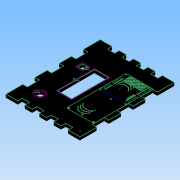
# Autodesk Inventor part: LCDWall
Saved by Autodesk Inventor 2015 (Build 190159000, 159)
## iProperties
Created: 2014-11-11
Part Number: LCDWall
Material: Generic
Document SubType Name: Modeling
Designer: 0
Density: 1 g/cm^3
Appearance: Plywood - Weathered
Mass: 139.736 g
Surface Area: 525.879 cm^2
Volume: 139.736 cm^3
Author: 0
Autodesk Inventor part; units mm, degrees
(part 1 of 2)
ref_plane "YZ Plane" through (0, 0, 0) normal (1, 0, 0) x (0, 1, 0)
ref_plane "XZ Plane" through (0, 0, 0) normal (0, 1, 0) x (-1, 0, 0)
ref_plane "XY Plane" through (0, 0, 0) normal (0, 0, 1) x (1, 0, 0)
sketch "Sketch1" plane through (0, 0, 0) normal (0, 1, 0) x (-1, 0, 0)
  line L0 (0, 0) -> (127, 0)
  line L1 (127, 0) -> (127, -166.624)
  line L2 (127, -166.624) -> (0, -166.624)
  line L3 (0, -166.624) -> (0, 0)
  dimension "BoxHeight" = 127
  dimension "d1" = 166.624
  constraints: 8 end point, 2 parallel, 1 coincident, 1 horizontal, 1 perpendicular
  measures "BoxHeight" distance of L1.end L2.end
  measures "d1" distance of L0.end L1.end
sketch "Sketch2" plane through (0, 0, 0) normal (0, 1, 0) x (-1, 0, 0)
  line L0 (0, 0) -> (-8.89, 0)
  line L1 (-8.89, 0) -> (-8.89, -23.8034)
  line L2 (-8.89, -23.8034) -> (0, -23.8034)
  line L3 (0, -23.8034) -> (0, 0)
  line L4 (0, -166.624) -> (0, 0) projected
  line L5 (0, 0) -> (127, 0) projected
  line L6 (0, -47.6069) -> (-8.89, -47.6069)
  line L7 (-8.89, -47.6069) -> (-8.89, -71.4103)
  line L8 (-8.89, -71.4103) -> (0, -71.4103)
  line L9 (0, -71.4103) -> (0, -47.6069)
  line L10 (0, -95.2137) -> (-8.89, -95.2137)
  line L11 (-8.89, -95.2137) -> (-8.89, -119.0171)
  line L12 (-8.89, -119.0171) -> (0, -119.0171)
  line L13 (0, -119.0171) -> (0, -95.2137)
  line L14 (63.5, 0) -> (63.5, -115.824) construction
  line L15 (127, -23.8034) -> (127, 0)
  line L16 (127, -166.624) -> (127, 0)
  line L17 (127, -71.4103) -> (127, -47.6069)
  line L18 (127, -119.0171) -> (127, -95.2137)
  line L19 (28.2222, -166.624) -> (14.1111, -166.624)
  line L20 (14.1111, -166.624) -> (14.1111, -175.514)
  line L21 (14.1111, -175.514) -> (28.2222, -175.514)
  line L22 (28.2222, -175.514) -> (28.2222, -166.624)
  line L23 (127, -166.624) -> (0, -166.624) projected
  line L24 (56.4444, -166.624) -> (42.3333, -166.624)
  line L25 (42.3333, -166.624) -> (42.3333, -175.514)
  line L26 (42.3333, -175.514) -> (56.4444, -175.514)
  line L27 (56.4444, -175.514) -> (56.4444, -166.624)
  line L28 (84.6667, -166.624) -> (70.5556, -166.624)
  line L29 (70.5556, -166.624) -> (70.5556, -175.514)
  line L30 (70.5556, -175.514) -> (84.6667, -175.514)
  line L31 (84.6667, -175.514) -> (84.6667, -166.624)
  line L32 (112.8889, -166.624) -> (98.7778, -166.624)
  line L33 (98.7778, -166.624) -> (98.7778, -175.514)
  line L34 (98.7778, -175.514) -> (112.8889, -175.514)
  line L35 (112.8889, -175.514) -> (112.8889, -166.624)
  line L36 (127, -83.312) -> (0, -83.312) construction
  line L37 (63.5, -166.624) -> (63.5, -50.8) construction
  line L38 (28.2222, 0) -> (14.1111, 0)
  line L39 (14.1111, 0) -> (14.1111, 8.89)
  line L40 (14.1111, 8.89) -> (28.2222, 8.89)
  line L41 (28.2222, 8.89) -> (28.2222, 0)
  line L42 (127, 0) -> (0, 0)
  line L43 (56.4444, 0) -> (42.3333, 0)
  line L44 (42.3333, 0) -> (42.3333, 8.89)
  line L45 (42.3333, 8.89) -> (56.4444, 8.89)
  line L46 (56.4444, 8.89) -> (56.4444, 0)
  line L47 (84.6667, 0) -> (70.5556, 0)
  line L48 (70.5556, 0) -> (70.5556, 8.89)
  line L49 (84.6667, 8.89) -> (84.6667, 0)
  line L50 (70.5556, 8.89) -> (84.6667, 8.89)
  line L51 (112.8889, 0) -> (98.7778, 0)
  line L52 (98.7778, 0) -> (98.7778, 8.89)
  line L53 (112.8889, 8.89) -> (112.8889, 0)
  line L54 (98.7778, 8.89) -> (112.8889, 8.89)
  line L55 (0, -142.8206) -> (-8.89, -142.8206)
  line L56 (-8.89, -142.8206) -> (-8.89, -159.3669)
  line L57 (-8.89, -159.3669) -> (0, -159.3669)
  line L58 (0, -159.3669) -> (0, -142.8206)
  line L59 (127, -166.624) -> (127, 0)
  line L60 (127, 0) -> (135.89, 0)
  line L61 (135.89, 0) -> (135.89, -23.8034)
  line L62 (135.89, -23.8034) -> (127, -23.8034)
  line L63 (127, -23.8034) -> (127, 0)
  line L64 (127, -166.624) -> (127, 0)
  line L65 (127, -47.6069) -> (135.89, -47.6069)
  line L66 (135.89, -47.6069) -> (135.89, -71.4103)
  line L67 (135.89, -71.4103) -> (127, -71.4103)
  line L68 (127, -71.4103) -> (127, -47.6069)
  line L69 (127, -95.2137) -> (135.89, -95.2137)
  line L70 (135.89, -95.2137) -> (135.89, -119.0171)
  line L71 (135.89, -119.0171) -> (127, -119.0171)
  line L72 (127, -119.0171) -> (127, -95.2137)
  line L73 (135.89, -142.8206) -> (135.89, -159.3669)
  line L74 (127, -142.8206) -> (135.89, -142.8206)
  line L75 (127, -159.3669) -> (127, -142.8206)
  line L76 (135.89, -159.3669) -> (127, -159.3669)
  line L77 (14.1111, -175.514) -> (0, -175.514)
  line L78 (0, -175.514) -> (0, -159.3669)
  line L79 (0, -159.3669) -> (14.1111, -159.3669)
  line L80 (14.1111, -159.3669) -> (14.1111, -175.514)
  line L81 (28.2222, -175.514) -> (42.3333, -175.514)
  line L82 (42.3333, -175.514) -> (42.3333, -166.624)
  line L83 (42.3333, -166.624) -> (28.2222, -166.624)
  line L84 (28.2222, -166.624) -> (28.2222, -175.514)
  line L85 (56.4444, -175.514) -> (70.5556, -175.514)
  line L86 (70.5556, -175.514) -> (70.5556, -166.624)
  line L87 (70.5556, -166.624) -> (56.4444, -166.624)
  line L88 (56.4444, -166.624) -> (56.4444, -175.514)
  line L89 (84.6667, -175.514) -> (98.7778, -175.514)
  line L90 (98.7778, -175.514) -> (98.7778, -166.624)
  line L91 (98.7778, -166.624) -> (84.6667, -166.624)
  line L92 (84.6667, -166.624) -> (84.6667, -175.514)
  line L93 (112.8889, -175.514) -> (127, -175.514)
  line L94 (127, -175.514) -> (127, -159.3669)
  line L95 (127, -159.3669) -> (112.8889, -159.3669)
  line L96 (112.8889, -159.3669) -> (112.8889, -175.514)
  line L97 (112.8889, 0) -> (127, 0)
  line L98 (127, 0) -> (127, 8.89)
  line L99 (127, 8.89) -> (112.8889, 8.89)
  line L100 (112.8889, 8.89) -> (112.8889, 0)
  line L101 (98.7778, 8.89) -> (84.6667, 8.89)
  line L102 (84.6667, 8.89) -> (84.6667, 0)
  line L103 (84.6667, 0) -> (98.7778, 0)
  line L104 (98.7778, 0) -> (98.7778, 8.89)
  line L105 (70.5556, 8.89) -> (56.4444, 8.89)
  line L106 (56.4444, 8.89) -> (56.4444, 0)
  line L107 (56.4444, 0) -> (70.5556, 0)
  line L108 (70.5556, 0) -> (70.5556, 8.89)
  line L109 (42.3333, 8.89) -> (28.2222, 8.89)
  line L110 (28.2222, 8.89) -> (28.2222, 0)
  line L111 (28.2222, 0) -> (42.3333, 0)
  line L112 (42.3333, 0) -> (42.3333, 8.89)
  line L113 (14.1111, 8.89) -> (0, 8.89)
  line L114 (0, 8.89) -> (0, 0)
  line L115 (0, 0) -> (14.1111, 0)
  line L116 (14.1111, 0) -> (14.1111, 8.89)
  line L117 (0, 0) -> (-8.89, 0)
  line L118 (-8.89, 0) -> (-8.89, 8.89)
  line L119 (-8.89, 8.89) -> (0, 8.89)
  line L120 (0, 8.89) -> (0, 0)
  line L121 (0, -159.3669) -> (-8.89, -159.3669)
  line L122 (-8.89, -159.3669) -> (-8.89, -168.2569)
  line L123 (-8.89, -168.2569) -> (0, -168.2569)
  line L124 (0, -168.2569) -> (0, -159.3669)
  line L125 (127, -159.3669) -> (135.89, -159.3669)
  line L126 (135.89, -159.3669) -> (135.89, -168.2569)
  line L127 (135.89, -168.2569) -> (127, -168.2569)
  line L128 (127, -168.2569) -> (127, -159.3669)
  line L129 (127, 0) -> (135.89, 0)
  line L130 (135.89, 0) -> (135.89, 8.89)
  line L131 (135.89, 8.89) -> (127, 8.89)
  line L132 (127, 8.89) -> (127, 0)
  line L133 (135.89, -168.2569) -> (127, -168.2569)
  line L134 (127, -168.2569) -> (127, -175.514)
  line L135 (127, -175.514) -> (135.89, -175.514)
  line L136 (135.89, -175.514) -> (135.89, -168.2569)
  line L137 (0, -175.514) -> (-8.89, -175.514)
  line L138 (-8.89, -175.514) -> (-8.89, -168.2569)
  line L139 (-8.89, -168.2569) -> (0, -168.2569)
  line L140 (0, -168.2569) -> (0, -175.514)
  dimension "d2" = 8.89
  dimension "d3" = 23.8034
  dimension "d5" = 8.89
  dimension "d6" = 23.8034
  dimension "d7" = 23.8034
  dimension "d8" = 8.89
  dimension "d9" = 23.8034
  dimension "d10" = 23.8034
  dimension "d11" = 14.1111
  dimension "d12" = 127
  dimension "d13" = 14.1111
  dimension "d14" = 8.89
  dimension "d15" = 8.89
  dimension "d16" = 14.1111
  dimension "d17" = 8.89
  dimension "d18" = 14.1111
  dimension "d22" = 8.89
  dimension "d23" = 14.1111
  dimension "d27" = 14.1111
  dimension "d28" = 14.1111
  dimension "d29" = 14.1111
  dimension "d34" = 8.89
  dimension "d35" = 16.5463
  dimension "d40" = 23.8034
  dimension "d41" = 8.89
  dimension "d42" = 8.89
  dimension "d43" = 8.89
  dimension "d44" = 8.89
  dimension "d45" = 8.89
  dimension "d46" = 8.89
  dimension "d47" = 8.89
  dimension "d48" = 8.89
  constraints: 276 end point, 48 parallel, 43 symmetric about line, 24 horizontal, 24 perpendicular, 9 collinear, 2 midpoint, 1 point on line, 1 vertical
  measures "d2" distance of L1.end L2.end
  measures "d3" distance of L0.end L1.end
  measures "d5" distance of L7.end L8.end
  measures "d6" distance of L6.end L7.end
  measures "d7" distance between parallel lines of L2 L6
  measures "d8" distance of L10.start L10.end
  measures "d9" distance of L10.end L11.end
  measures "d10" distance between parallel lines of L8 L10
  measures "d11" distance between parallel lines of L4 L20
  measures "d12" distance of L23.start L4.start
  measures "d13" distance of L20.end L21.end
  measures "d14" distance of L19.end L20.end
  measures "d15" distance of L24.end L25.end
  measures "d16" distance of L25.end L26.end
  measures "d17" distance of L28.end L29.end
  measures "d18" distance of L29.end L31.start
  measures "d22" distance of L32.end L33.end
  measures "d23" distance of L33.end L35.start
  measures "d27" distance between parallel lines of L25 L22
  measures "d28" distance between parallel lines of L27 L29
  measures "d29" distance between parallel lines of L31 L33
  measures "d34" distance of L55.start L56.start
  measures "d35" distance of L56.start L56.end
  measures "d40" distance between parallel lines of L12 L55
  measures "d41" distance of L118.end L119.end
  measures "d42" distance of L117.end L118.end
  measures "d43" distance of L123.end L122.end
  measures "d44" distance of L122.end L121.end
  measures "d45" distance of L126.end L127.end
  measures "d46" distance of L125.end L126.end
  measures "d47" distance of L131.end L130.end
  measures "d48" distance of L130.end L129.end
extrude "Connections" add sketch "Sketch2" along normal blind 6.35 contours L3 L2 L1 L0 | L114 L113 L39 L5 | L0 L118 L119 L114 | L4 L8 L7 L6 | L41 L109 L44 L5 | L4 L12 L11 L10 | L46 L105 L48 L5 | L4 L57 L56 L55 | L49 L101 L52 L5 | L79 L80 L23 L4 | L4 L78 L123 L122 L57 | L23 L20 L77 L78 | L53 L99 L98 L5 | L78 L137 L138 L123 | L60 L61 L62 L15 | L98 L131 L130 L60 | L23 L25 L81 L22 | L65 L66 L67 L16 | L23 L29 L85 L27 | L69 L70 L71 L16 | L23 L33 L89 L31 | L74 L73 L76 L16 | L96 L95 L16 L23 | L23 L94 L93 L35 | L76 L126 L127 L94 L16 | L94 L127 L136 L135
extrude "Base Extrusion" add sketch "Sketch1" along normal blind 6.35
sketch "Sketch3" plane through (0, 0, 0) normal (0, -1, 0) x (1, 0, 0)
  line L0 (-70.5556, 8.89) -> (-56.4444, 8.89) projected
  line L1 (-63.5, 8.89) -> (-63.5, -175.514) construction
  line L2 (-56.4444, -175.514) -> (-70.5556, -175.514) projected
  line L3 (8.89, -83.312) -> (-135.89, -83.312) construction
  line L4 (-28.2222, -175.514) -> (-42.3333, -175.514) projected
  line L5 (-42.3333, 8.89) -> (-28.2222, 8.89) projected
  line L6 (8.89, -175.514) -> (8.89, -142.8206) projected
  line L7 (-135.89, -175.514) -> (-135.89, -142.8206) projected
  line L8 (-135.89, -119.0171) -> (-135.89, -95.2137) projected
  line L9 (-91.186, -47.117) -> (-63.5, -47.117)
  line L10 (-63.5, -47.117) -> (-63.5, -119.507)
  line L11 (-63.5, -119.507) -> (-91.186, -119.507)
  line L12 (-91.186, -119.507) -> (-91.186, -47.117)
  point P0 (0, 0)
  point P1 (8.89, -168.2569)
  point P2 (-135.89, -168.2569)
  dimension "d49" = 184.404
  dimension "d50" = 92.202
  dimension "d51" = 144.78
  dimension "d52" = 144.78
  dimension "d53" = 0
  dimension "d54" = 27.686
  dimension "d55" = 72.39
  dimension "d56" = 27.686
  dimension "d57" = 36.195
  constraints: 12 end point, 2 horizontal, 2 midpoint, 2 parallel, 1 perpendicular
  measures "d49" distance between parallel lines of L4 L5
  measures "d50" distance between parallel lines of L4 L3
  measures "d51" distance between parallel lines of L6 L7
  measures "d52" distance of L3.start L3.end
  measures "d53" distance from line of L8 L3.end
  measures "d54" distance of L10.end L11.end
  measures "d55" distance of L11.end L9.start
  measures "d56" distance between parallel lines of L1 L12
  measures "d57" distance between parallel lines of L3 L9
extrude "LCD Hole" cut sketch "Sketch3" against normal blind 25.4
sketch "Sketch5" plane through (0, 0, 0) normal (0, -1, 0) x (1, 0, 0)
  line L0 (-3.8506, -48.6761) -> (-3.8506, -68.028) construction
  line L1 (-3.8506, -68.028) -> (-44.1343, -68.028) construction
  line L2 (-44.1343, -68.028) -> (-44.1343, -48.6761) construction
  line L3 (-44.1343, -48.6761) -> (-3.8506, -48.6761) construction
  point P0 (0, 0)
  constraints: 2 other
sketch "Sketch7" plane through (0, 6.35, 0) normal (0, 1, 0) x (1, 0, 0)
  circle A0 centre (-102.8514, 25.0329) radius 6.985 projected
  point P0 (0, 0)
extrude "Extrusion4" cut sketch "Sketch7" against normal blind 25.4
sketch "Sketch6" plane through (0, 6.35, 0) normal (0, 1, 0) x (1, 0, 0)
  arc A0 (-44.8569, 41.3319) -> (-21.0385, 41.4572) centre (-32.9709, 45.8056) ccw
  arc A1 (-44.9033, 46.638) -> (-21.0849, 46.5126) centre (-32.9709, 50.9863) ccw
  arc A2 (-44.8569, 51.4366) -> (-21.0849, 51.4366) centre (-32.9709, 55.9103) ccw
  line L0 (-21.0385, 41.4572) -> (-44.9033, 41.4572) construction
  line L1 (-44.9033, 41.4572) -> (-44.9033, 76.962) construction
  line L2 (-44.9033, 76.962) -> (-21.0385, 76.962) construction
  line L3 (-21.0385, 76.962) -> (-21.0385, 41.4572) construction
  line L4 (-63.5, 47.117) -> (-2.4418, 47.117) construction
  line L5 (-2.4418, 47.117) -> (-2.4418, 119.507) construction
  line L6 (-2.4418, 119.507) -> (-63.5, 119.507) construction
  line L7 (-63.5, 119.507) -> (-63.5, 47.117) construction
  line L8 (-2.4418, 83.312) -> (-63.5, 83.312) construction
  line L9 (-63.5, 47.117) -> (-63.5, 119.507) projected
  line L10 (-32.9709, 47.117) -> (-32.9709, 119.507) construction
  line L11 (-46.2663, 76.962) -> (-23.7437, 76.962) construction
  line L12 (-21.5465, 41.5479) -> (-21.5465, 51.054) construction
  arc A3 (-44.3611, 46.638) -> (-21.6293, 46.5126) centre (-32.9709, 50.9863) ccw
  arc A4 (-44.3125, 51.4366) -> (-21.6293, 51.4366) centre (-32.9709, 55.9103) ccw
  line L13 (-21.5465, 51.054) -> (-21.5465, 41.5479) construction
  line L14 (-44.8569, 41.3319) -> (-44.3125, 41.3319)
  arc A5 (-44.3125, 41.3319) -> (-21.5807, 41.4572) centre (-32.9709, 45.8056) ccw
  line L15 (-21.0385, 41.4572) -> (-21.5807, 41.4572)
  line L16 (-21.0849, 46.5126) -> (-21.6293, 46.5126)
  line L17 (-21.0849, 51.4366) -> (-21.6293, 51.4366)
  line L18 (-44.9033, 46.638) -> (-44.3611, 46.638)
  line L19 (-44.3611, 76.962) -> (-44.9033, 76.962)
  line L20 (-21.6293, 51.4366) -> (4.4309, 51.4366) construction
  line L21 (-44.3125, 51.4366) -> (-44.8569, 51.4366)
  arc A6 (-21.0385, 125.1668) -> (-44.8569, 125.2921) centre (-32.9709, 120.8184) ccw
  arc A7 (-21.0849, 120.1114) -> (-44.9033, 119.986) centre (-32.9709, 115.6377) ccw
  arc A8 (-21.0849, 115.1874) -> (-44.8569, 115.1874) centre (-32.9709, 110.7137) ccw
  line L22 (-21.0385, 125.1668) -> (-44.9033, 125.1668) construction
  line L23 (-44.9033, 125.1668) -> (-44.9033, 89.662) construction
  line L24 (-44.9033, 89.662) -> (-21.0385, 89.662) construction
  line L25 (-21.0385, 89.662) -> (-21.0385, 125.1668) construction
  line L26 (-32.9709, 119.507) -> (-32.9709, 47.117) construction
  line L27 (-46.2663, 89.662) -> (-23.7437, 89.662) construction
  line L28 (-21.5465, 125.0761) -> (-21.5465, 115.57) construction
  arc A9 (-21.6293, 120.1114) -> (-44.3611, 119.986) centre (-32.9709, 115.6377) ccw
  arc A10 (-21.6293, 115.1874) -> (-44.3125, 115.1874) centre (-32.9709, 110.7137) ccw
  line L29 (-21.5465, 115.57) -> (-21.5465, 125.0761) construction
  line L30 (-44.8569, 125.2921) -> (-44.3125, 125.2921)
  arc A11 (-21.5807, 125.1668) -> (-44.3125, 125.2921) centre (-32.9709, 120.8184) ccw
  line L31 (-21.0385, 125.1668) -> (-21.5807, 125.1668)
  line L32 (-21.0849, 120.1114) -> (-21.6293, 120.1114)
  line L33 (-21.0849, 115.1874) -> (-21.6293, 115.1874)
  line L34 (-44.9033, 119.986) -> (-44.3611, 119.986)
  line L35 (-44.3611, 89.662) -> (-44.9033, 89.662)
  line L36 (-21.6293, 115.1874) -> (4.4309, 115.1874) construction
  line L37 (-44.3125, 115.1874) -> (-44.8569, 115.1874)
  line L38 (-0.1825, 29.2815) -> (-0.1825, 141.0415) projected
  arc A12 (-2.7225, 26.7415) -> (-0.1825, 29.2815) centre (-2.7225, 29.2815) ccw projected
  line L39 (-50.9825, 26.7415) -> (-2.7225, 26.7415) projected
  arc A13 (-53.5225, 29.2815) -> (-50.9825, 26.7415) centre (-50.9825, 29.2815) ccw projected
  line L40 (-53.5225, 141.0415) -> (-53.5225, 29.2815) projected
  arc A14 (-50.9825, 143.5815) -> (-53.5225, 141.0415) centre (-50.9825, 141.0415) ccw projected
  line L41 (-2.7225, 143.5815) -> (-50.9825, 143.5815) projected
  arc A15 (-0.1825, 141.0415) -> (-2.7225, 143.5815) centre (-2.7225, 141.0415) ccw projected
  line L42 (-2.405, 141.994) -> (-2.405, 141.359) projected
  line L43 (-3.04, 141.994) -> (-2.405, 141.994) projected
  line L44 (-3.04, 141.359) -> (-3.04, 141.994) projected
  line L45 (-2.405, 141.359) -> (-3.04, 141.359) projected
  line L46 (-50.665, 127.389) -> (-50.665, 126.754) projected
  line L47 (-51.3, 127.389) -> (-50.665, 127.389) projected
  line L48 (-51.3, 126.754) -> (-51.3, 127.389) projected
  line L49 (-50.665, 126.754) -> (-51.3, 126.754) projected
  line L50 (-50.665, 122.309) -> (-50.665, 121.674) projected
  line L51 (-51.3, 122.309) -> (-50.665, 122.309) projected
  line L52 (-51.3, 121.674) -> (-51.3, 122.309) projected
  line L53 (-50.665, 121.674) -> (-51.3, 121.674) projected
  line L54 (-50.665, 117.229) -> (-50.665, 116.594) projected
  line L55 (-51.3, 117.229) -> (-50.665, 117.229) projected
  line L56 (-51.3, 116.594) -> (-51.3, 117.229) projected
  line L57 (-50.665, 116.594) -> (-51.3, 116.594) projected
  line L58 (-50.665, 109.609) -> (-50.665, 108.974) projected
  line L59 (-51.3, 109.609) -> (-50.665, 109.609) projected
  line L60 (-51.3, 108.974) -> (-51.3, 109.609) projected
  line L61 (-50.665, 108.974) -> (-51.3, 108.974) projected
  line L62 (-50.665, 104.529) -> (-50.665, 103.894) projected
  line L63 (-51.3, 104.529) -> (-50.665, 104.529) projected
  line L64 (-51.3, 103.894) -> (-51.3, 104.529) projected
  line L65 (-50.665, 103.894) -> (-51.3, 103.894) projected
  line L66 (-50.665, 99.449) -> (-50.665, 98.814) projected
  line L67 (-51.3, 99.449) -> (-50.665, 99.449) projected
  line L68 (-51.3, 98.814) -> (-51.3, 99.449) projected
  line L69 (-50.665, 98.814) -> (-51.3, 98.814) projected
  line L70 (-2.405, 115.324) -> (-2.405, 114.689) projected
  line L71 (-3.04, 115.324) -> (-2.405, 115.324) projected
  line L72 (-3.04, 114.689) -> (-3.04, 115.324) projected
  line L73 (-2.405, 114.689) -> (-3.04, 114.689) projected
  line L74 (-3.04, 136.914) -> (-2.405, 136.914) projected
  line L75 (-3.04, 136.279) -> (-3.04, 136.914) projected
  line L76 (-2.405, 136.279) -> (-3.04, 136.279) projected
  line L77 (-2.405, 136.914) -> (-2.405, 136.279) projected
  line L78 (-3.04, 131.834) -> (-2.405, 131.834) projected
  line L79 (-3.04, 131.199) -> (-3.04, 131.834) projected
  line L80 (-2.405, 131.199) -> (-3.04, 131.199) projected
  line L81 (-2.405, 131.834) -> (-2.405, 131.199) projected
  line L82 (-3.04, 126.754) -> (-2.405, 126.754) projected
  line L83 (-3.04, 126.119) -> (-3.04, 126.754) projected
  line L84 (-2.405, 126.119) -> (-3.04, 126.119) projected
  line L85 (-2.405, 126.754) -> (-2.405, 126.119) projected
  line L86 (-3.04, 121.674) -> (-2.405, 121.674) projected
  line L87 (-3.04, 121.039) -> (-3.04, 121.674) projected
  line L88 (-2.405, 121.039) -> (-3.04, 121.039) projected
  line L89 (-2.405, 121.674) -> (-2.405, 121.039) projected
  line L90 (-2.405, 112.784) -> (-2.405, 112.149) projected
  line L91 (-3.04, 112.784) -> (-2.405, 112.784) projected
  line L92 (-3.04, 112.149) -> (-3.04, 112.784) projected
  line L93 (-2.405, 112.149) -> (-3.04, 112.149) projected
  line L94 (-2.405, 107.704) -> (-2.405, 107.069) projected
  line L95 (-3.04, 107.704) -> (-2.405, 107.704) projected
  line L96 (-3.04, 107.069) -> (-3.04, 107.704) projected
  line L97 (-2.405, 107.069) -> (-3.04, 107.069) projected
  line L98 (-2.405, 102.624) -> (-2.405, 101.989) projected
  line L99 (-3.04, 102.624) -> (-2.405, 102.624) projected
  line L100 (-3.04, 101.989) -> (-3.04, 102.624) projected
  line L101 (-2.405, 101.989) -> (-3.04, 101.989) projected
  line L102 (-2.405, 97.544) -> (-2.405, 96.909) projected
  line L103 (-3.04, 97.544) -> (-2.405, 97.544) projected
  line L104 (-3.04, 96.909) -> (-3.04, 97.544) projected
  line L105 (-2.405, 96.909) -> (-3.04, 96.909) projected
  circle A16 centre (-9.0725, 102.3065) radius 0.635 projected
  circle A17 centre (-9.0725, 104.8465) radius 0.635 projected
  circle A18 centre (-9.0725, 107.3865) radius 0.635 projected
  circle A19 centre (-9.0725, 109.9265) radius 0.635 projected
  circle A20 centre (-9.0725, 112.4665) radius 0.635 projected
  circle A21 centre (-9.0725, 115.0065) radius 0.635 projected
  circle A22 centre (-24.884, 29.9165) radius 0.3175 projected
  circle A23 centre (-26.535, 30.9325) radius 0.3175 projected
  circle A24 centre (-26.535, 32.9645) radius 0.3175 projected
  circle A25 centre (-23.36, 85.0345) radius 0.3175 projected
  circle A26 centre (-26.535, 86.0505) radius 0.3175 projected
  line L106 (-2.405, 100.084) -> (-2.405, 99.449) projected
  line L107 (-3.04, 100.084) -> (-2.405, 100.084) projected
  line L108 (-3.04, 99.449) -> (-3.04, 100.084) projected
  line L109 (-2.405, 99.449) -> (-3.04, 99.449) projected
  line L110 (-2.405, 105.164) -> (-2.405, 104.529) projected
  line L111 (-3.04, 105.164) -> (-2.405, 105.164) projected
  line L112 (-3.04, 104.529) -> (-3.04, 105.164) projected
  line L113 (-2.405, 104.529) -> (-3.04, 104.529) projected
  line L114 (-2.405, 110.244) -> (-2.405, 109.609) projected
  line L115 (-3.04, 110.244) -> (-2.405, 110.244) projected
  line L116 (-3.04, 109.609) -> (-3.04, 110.244) projected
  line L117 (-2.405, 109.609) -> (-3.04, 109.609) projected
  line L118 (-3.04, 119.134) -> (-2.405, 119.134) projected
  line L119 (-3.04, 118.499) -> (-3.04, 119.134) projected
  line L120 (-2.405, 118.499) -> (-3.04, 118.499) projected
  line L121 (-2.405, 119.134) -> (-2.405, 118.499) projected
  line L122 (-3.04, 124.214) -> (-2.405, 124.214) projected
  line L123 (-3.04, 123.579) -> (-3.04, 124.214) projected
  line L124 (-2.405, 123.579) -> (-3.04, 123.579) projected
  line L125 (-2.405, 124.214) -> (-2.405, 123.579) projected
  line L126 (-3.04, 129.294) -> (-2.405, 129.294) projected
  line L127 (-3.04, 128.659) -> (-3.04, 129.294) projected
  line L128 (-2.405, 128.659) -> (-3.04, 128.659) projected
  line L129 (-2.405, 129.294) -> (-2.405, 128.659) projected
  line L130 (-3.04, 134.374) -> (-2.405, 134.374) projected
  line L131 (-3.04, 133.739) -> (-3.04, 134.374) projected
  line L132 (-2.405, 133.739) -> (-3.04, 133.739) projected
  line L133 (-2.405, 134.374) -> (-2.405, 133.739) projected
  line L134 (-3.04, 139.454) -> (-2.405, 139.454) projected
  line L135 (-3.04, 138.819) -> (-3.04, 139.454) projected
  line L136 (-2.405, 138.819) -> (-3.04, 138.819) projected
  line L137 (-2.405, 139.454) -> (-2.405, 138.819) projected
  line L138 (-50.665, 96.909) -> (-50.665, 96.274) projected
  line L139 (-51.3, 96.909) -> (-50.665, 96.909) projected
  line L140 (-51.3, 96.274) -> (-51.3, 96.909) projected
  line L141 (-50.665, 96.274) -> (-51.3, 96.274) projected
  line L142 (-50.665, 101.989) -> (-50.665, 101.354) projected
  line L143 (-51.3, 101.989) -> (-50.665, 101.989) projected
  line L144 (-51.3, 101.354) -> (-51.3, 101.989) projected
  line L145 (-50.665, 101.354) -> (-51.3, 101.354) projected
  line L146 (-50.665, 107.069) -> (-50.665, 106.434) projected
  line L147 (-51.3, 107.069) -> (-50.665, 107.069) projected
  line L148 (-51.3, 106.434) -> (-51.3, 107.069) projected
  line L149 (-50.665, 106.434) -> (-51.3, 106.434) projected
  line L150 (-50.665, 114.689) -> (-50.665, 114.054) projected
  line L151 (-51.3, 114.689) -> (-50.665, 114.689) projected
  line L152 (-51.3, 114.054) -> (-51.3, 114.689) projected
  line L153 (-50.665, 114.054) -> (-51.3, 114.054) projected
  line L154 (-50.665, 119.769) -> (-50.665, 119.134) projected
  line L155 (-51.3, 119.769) -> (-50.665, 119.769) projected
  line L156 (-51.3, 119.134) -> (-51.3, 119.769) projected
  line L157 (-50.665, 119.134) -> (-51.3, 119.134) projected
  line L158 (-50.665, 124.849) -> (-50.665, 124.214) projected
  line L159 (-51.3, 124.849) -> (-50.665, 124.849) projected
  line L160 (-51.3, 124.214) -> (-51.3, 124.849) projected
  line L161 (-50.665, 124.214) -> (-51.3, 124.214) projected
  line L162 (-50.665, 129.929) -> (-50.665, 129.294) projected
  line L163 (-51.3, 129.929) -> (-50.665, 129.929) projected
  line L164 (-51.3, 129.294) -> (-51.3, 129.929) projected
  line L165 (-50.665, 129.294) -> (-51.3, 129.294) projected
  line L166 (-50.665, 132.469) -> (-50.665, 131.834) projected
  line L167 (-51.3, 132.469) -> (-50.665, 132.469) projected
  line L168 (-51.3, 131.834) -> (-51.3, 132.469) projected
  line L169 (-50.665, 131.834) -> (-51.3, 131.834) projected
  circle A27 centre (-47.1725, 96.5915) radius 0.635 projected
  circle A28 centre (-47.1725, 99.1315) radius 0.635 projected
  circle A29 centre (-47.1725, 101.6715) radius 0.635 projected
  circle A30 centre (-47.1725, 104.2115) radius 0.635 projected
  circle A31 centre (-47.1725, 106.7515) radius 0.635 projected
  circle A32 centre (-47.1725, 109.2915) radius 0.635 projected
  circle A33 centre (-47.1725, 114.3715) radius 0.635 projected
  circle A34 centre (-47.1725, 116.9115) radius 0.635 projected
  circle A35 centre (-47.1725, 119.4515) radius 0.635 projected
  circle A36 centre (-47.1725, 121.9915) radius 0.635 projected
  circle A37 centre (-47.1725, 124.5315) radius 0.635 projected
  circle A38 centre (-47.1725, 127.0715) radius 0.635 projected
  circle A39 centre (-47.1725, 129.6115) radius 0.635 projected
  circle A40 centre (-47.1725, 132.1515) radius 0.635 projected
  circle A41 centre (-6.5325, 97.2265) radius 0.635 projected
  circle A42 centre (-6.5325, 99.7665) radius 0.635 projected
  circle A43 centre (-6.5325, 102.3065) radius 0.635 projected
  circle A44 centre (-6.5325, 104.8465) radius 0.635 projected
  circle A45 centre (-6.5325, 107.3865) radius 0.635 projected
  circle A46 centre (-6.5325, 109.9265) radius 0.635 projected
  circle A47 centre (-6.5325, 112.4665) radius 0.635 projected
  circle A48 centre (-6.5325, 118.8165) radius 0.635 projected
  circle A49 centre (-6.5325, 121.3565) radius 0.635 projected
  circle A50 centre (-6.5325, 123.8965) radius 0.635 projected
  circle A51 centre (-6.5325, 126.4365) radius 0.635 projected
  circle A52 centre (-6.5325, 128.9765) radius 0.635 projected
  circle A53 centre (-6.5325, 131.5165) radius 0.635 projected
  circle A54 centre (-6.5325, 134.0565) radius 0.635 projected
  circle A55 centre (-6.5325, 136.5965) radius 0.635 projected
  circle A56 centre (-6.5325, 139.1365) radius 0.635 projected
  circle A57 centre (-6.5325, 115.0065) radius 0.635 projected
  circle A58 centre (-6.5325, 141.6765) radius 0.635 projected
  circle A59 centre (-10.3425, 141.6765) radius 0.635 projected
  circle A60 centre (-12.8825, 141.6765) radius 0.635 projected
  circle A61 centre (-15.4225, 141.6765) radius 0.635 projected
  circle A62 centre (-17.9625, 141.6765) radius 0.635 projected
  circle A63 centre (-20.5025, 141.6765) radius 0.635 projected
  circle A64 centre (-23.0425, 141.6765) radius 0.635 projected
  circle A65 centre (-25.5825, 141.6765) radius 0.635 projected
  circle A66 centre (-28.1225, 141.6765) radius 0.635 projected
  circle A67 centre (-30.6625, 141.6765) radius 0.635 projected
  circle A68 centre (-33.2025, 141.6765) radius 0.635 projected
  circle A69 centre (-35.7425, 141.6765) radius 0.635 projected
  circle A70 centre (-38.2825, 141.6765) radius 0.635 projected
  circle A71 centre (-40.8225, 141.6765) radius 0.635 projected
  circle A72 centre (-10.3425, 128.9765) radius 0.635 projected
  circle A73 centre (-10.3425, 131.5165) radius 0.635 projected
  circle A74 centre (-10.3425, 134.0565) radius 0.635 projected
  circle A75 centre (-10.3425, 136.5965) radius 0.635 projected
  circle A76 centre (-10.3425, 139.1365) radius 0.635 projected
  circle A77 centre (-12.8825, 128.9765) radius 0.635 projected
  circle A78 centre (-12.8825, 131.5165) radius 0.635 projected
  circle A79 centre (-12.8825, 134.0565) radius 0.635 projected
  circle A80 centre (-12.8825, 136.5965) radius 0.635 projected
  circle A81 centre (-12.8825, 139.1365) radius 0.635 projected
  circle A82 centre (-15.4225, 128.9765) radius 0.635 projected
  circle A83 centre (-15.4225, 131.5165) radius 0.635 projected
  circle A84 centre (-15.4225, 134.0565) radius 0.635 projected
  circle A85 centre (-15.4225, 136.5965) radius 0.635 projected
  circle A86 centre (-15.4225, 139.1365) radius 0.635 projected
  circle A87 centre (-17.9625, 128.9765) radius 0.635 projected
  circle A88 centre (-17.9625, 131.5165) radius 0.635 projected
  circle A89 centre (-17.9625, 134.0565) radius 0.635 projected
  circle A90 centre (-17.9625, 136.5965) radius 0.635 projected
  circle A91 centre (-17.9625, 139.1365) radius 0.635 projected
  circle A92 centre (-20.5025, 128.9765) radius 0.635 projected
  circle A93 centre (-20.5025, 131.5165) radius 0.635 projected
  circle A94 centre (-20.5025, 134.0565) radius 0.635 projected
  circle A95 centre (-20.5025, 136.5965) radius 0.635 projected
  circle A96 centre (-20.5025, 139.1365) radius 0.635 projected
  circle A97 centre (-23.0425, 128.9765) radius 0.635 projected
  circle A98 centre (-23.0425, 131.5165) radius 0.635 projected
  circle A99 centre (-23.0425, 134.0565) radius 0.635 projected
  circle A100 centre (-23.0425, 136.5965) radius 0.635 projected
  circle A101 centre (-23.0425, 139.1365) radius 0.635 projected
  circle A102 centre (-25.5825, 128.9765) radius 0.635 projected
  circle A103 centre (-25.5825, 131.5165) radius 0.635 projected
  circle A104 centre (-25.5825, 134.0565) radius 0.635 projected
  circle A105 centre (-25.5825, 136.5965) radius 0.635 projected
  circle A106 centre (-25.5825, 139.1365) radius 0.635 projected
  circle A107 centre (-28.1225, 128.9765) radius 0.635 projected
  circle A108 centre (-28.1225, 131.5165) radius 0.635 projected
  circle A109 centre (-28.1225, 134.0565) radius 0.635 projected
  circle A110 centre (-28.1225, 136.5965) radius 0.635 projected
  circle A111 centre (-28.1225, 139.1365) radius 0.635 projected
  circle A112 centre (-30.6625, 128.9765) radius 0.635 projected
  circle A113 centre (-30.6625, 131.5165) radius 0.635 projected
  circle A114 centre (-30.6625, 134.0565) radius 0.635 projected
  circle A115 centre (-30.6625, 136.5965) radius 0.635 projected
  circle A116 centre (-30.6625, 139.1365) radius 0.635 projected
  circle A117 centre (-33.2025, 128.9765) radius 0.635 projected
  circle A118 centre (-33.2025, 131.5165) radius 0.635 projected
  circle A119 centre (-33.2025, 134.0565) radius 0.635 projected
  circle A120 centre (-33.2025, 136.5965) radius 0.635 projected
  circle A121 centre (-33.2025, 139.1365) radius 0.635 projected
  circle A122 centre (-35.7425, 128.9765) radius 0.635 projected
  circle A123 centre (-35.7425, 131.5165) radius 0.635 projected
  circle A124 centre (-35.7425, 134.0565) radius 0.635 projected
  circle A125 centre (-35.7425, 136.5965) radius 0.635 projected
  circle A126 centre (-35.7425, 139.1365) radius 0.635 projected
  circle A127 centre (-38.2825, 128.9765) radius 0.635 projected
  circle A128 centre (-38.2825, 131.5165) radius 0.635 projected
  circle A129 centre (-38.2825, 134.0565) radius 0.635 projected
  circle A130 centre (-38.2825, 136.5965) radius 0.635 projected
  circle A131 centre (-38.2825, 139.1365) radius 0.635 projected
  circle A132 centre (-40.8225, 128.9765) radius 0.635 projected
  circle A133 centre (-40.8225, 131.5165) radius 0.635 projected
  circle A134 centre (-40.8225, 134.0565) radius 0.635 projected
  circle A135 centre (-40.8225, 136.5965) radius 0.635 projected
  circle A136 centre (-40.8225, 139.1365) radius 0.635 projected
  circle A137 centre (-43.3625, 128.9765) radius 0.635 projected
  circle A138 centre (-43.3625, 131.5165) radius 0.635 projected
  circle A139 centre (-43.3625, 134.0565) radius 0.635 projected
  circle A140 centre (-43.3625, 136.5965) radius 0.635 projected
  circle A141 centre (-43.3625, 139.1365) radius 0.635 projected
  circle A142 centre (-43.3625, 141.6765) radius 0.635 projected
  circle A143 centre (-50.9825, 29.2815) radius 1.5875 projected
  circle A144 centre (-50.9825, 91.5115) radius 1.5875 projected
  circle A145 centre (-2.7225, 91.5115) radius 1.5875 projected
  circle A146 centre (-2.7225, 29.2815) radius 1.5875 projected
  point P0 (0, 0)
  dimension "d60" = 12.7
  dimension "d61" = 12.7
  dimension "d62" = 12.7
  dimension "d63" = 6.35
  dimension "d65" = 0.508
  dimension "d66" = 0.508
  constraints: 74 end point, 29 symmetric about line, 26 point on circle, 12 centre point, 7 horizontal, 6 point on line, 5 parallel, 4 midpoint, 2 perpendicular, 1 collinear, 6 other
  measures "d60" radius of A0
  measures "d61" radius of A1
  measures "d62" radius of A2
  measures "d63" distance between parallel lines of L11 L8
  measures "d65" radial gap between concentric circles of A1 A3
  measures "d66" radial gap between concentric circles of A2 A4
emboss "Emboss1" sketch "Sketch6" operation cut depth 2.54 direction (0, -1, 0) picked at (-23.299, 128.7982) picked at (-27.8908, 131.9685) picked at (-25.7963, 131.1634) picked at (-38.4496, 131.8532) picked at (-33.2154, 133.4854) picked at (-40.4723, 131.0393) picked at (-42.945, 128.6155) contours L14 A5 L15 A0 | L18 A3 L16 A1 | L21 A4 L17 A2 | L31 A11 A108 A128 L30 A6 A137 A133 A119 A103 A97 | A97 A6 | A11 A108 | A103 A6 | A11 A128 | A119 A6 | A133 A6 | A6 A137 | L32 A9 L34 A7 | L33 A10 L37 A8
sketch "Sketch8" plane through (0, 6.35, 0) normal (0, 1, 0) x (1, 0, 0)
  line L0 (-112.555, 117.3994) -> (-112.555, 107.3994) projected
  line L1 (-112.555, 107.3994) -> (-102.555, 107.3994) projected
  line L2 (-102.555, 107.3994) -> (-102.555, 108.3994) projected
  line L3 (-103.055, 108.3994) -> (-103.055, 112.3994) projected
  line L4 (-102.555, 108.3994) -> (-103.055, 108.3994) projected
  line L5 (-103.055, 112.3994) -> (-103.055, 116.3994) projected
  line L6 (-102.555, 117.3994) -> (-112.555, 117.3994) projected
  line L7 (-103.055, 116.3994) -> (-102.555, 116.3994) projected
  line L8 (-102.555, 116.3994) -> (-102.555, 117.3994) projected
  circle A0 centre (-107.555, 112.3994) radius 4.25 projected
  circle A1 centre (-107.555, 112.3994) radius 4 projected
  circle A2 centre (-102.8514, 25.0329) radius 6.985 projected
  arc A3 (-21.0849, 120.1114) -> (-44.9033, 119.986) centre (-32.9709, 115.6377) ccw projected
  line L9 (-21.0849, 120.1114) -> (-21.6293, 120.1114) projected
  arc A4 (-21.6293, 120.1114) -> (-44.3611, 119.986) centre (-32.9709, 115.6377) ccw projected
  line L10 (-44.3611, 119.986) -> (-44.9033, 119.986) projected
  line L11 (-21.6293, 51.4366) -> (-21.0849, 51.4366) projected
  arc A5 (-44.8569, 51.4366) -> (-21.0849, 51.4366) centre (-32.9709, 55.9103) ccw projected
  line L12 (-44.8569, 51.4366) -> (-44.3125, 51.4366) projected
  arc A6 (-44.3125, 51.4366) -> (-21.6293, 51.4366) centre (-32.9709, 55.9103) ccw projected
  arc A7 (-21.0849, 115.1874) -> (-44.8569, 115.1874) centre (-32.9709, 110.7137) ccw projected
  line L13 (-21.0849, 115.1874) -> (-21.6293, 115.1874) projected
  arc A8 (-21.6293, 115.1874) -> (-44.3125, 115.1874) centre (-32.9709, 110.7137) ccw projected
  line L14 (-44.3125, 115.1874) -> (-44.8569, 115.1874) projected
  line L15 (-21.6293, 46.5126) -> (-21.0849, 46.5126) projected
  arc A9 (-44.9033, 46.638) -> (-21.0849, 46.5126) centre (-32.9709, 50.9863) ccw projected
  line L16 (-44.9033, 46.638) -> (-44.3611, 46.638) projected
  arc A10 (-44.3611, 46.638) -> (-21.6293, 46.5126) centre (-32.9709, 50.9863) ccw projected
  arc A11 (-44.8569, 41.3319) -> (-21.0385, 41.4572) centre (-32.9709, 45.8056) ccw projected
  line L17 (-44.8569, 41.3319) -> (-44.3125, 41.3319) projected
  arc A12 (-44.3125, 41.3319) -> (-21.5807, 41.4572) centre (-32.9709, 45.8056) ccw projected
  line L18 (-21.5807, 41.4572) -> (-21.0385, 41.4572) projected
  line L19 (-44.3125, 125.2921) -> (-44.8569, 125.2921) projected
  arc A13 (-21.0385, 125.1668) -> (-44.8569, 125.2921) centre (-32.9709, 120.8184) ccw projected
  line L20 (-21.0385, 125.1668) -> (-21.5807, 125.1668) projected
  arc A14 (-21.5807, 125.1668) -> (-44.3125, 125.2921) centre (-32.9709, 120.8184) ccw projected
  line L21 (-91.186, 47.117) -> (-91.186, 119.507) projected
  line L22 (-91.186, 119.507) -> (-63.5, 119.507) projected
  line L23 (-63.5, 119.507) -> (-63.5, 47.117) projected
  line L24 (-63.5, 47.117) -> (-91.186, 47.117) projected
  line L25 (-127, 119.0171) -> (-135.89, 119.0171) projected
  line L26 (-135.89, 119.0171) -> (-135.89, 95.2137) projected
  line L27 (-135.89, 95.2137) -> (-127, 95.2137) projected
  line L28 (-127, 95.2137) -> (-127, 71.4103) projected
  line L29 (-127, 71.4103) -> (-135.89, 71.4103) projected
  line L30 (-135.89, 71.4103) -> (-135.89, 47.6069) projected
  line L31 (-135.89, 47.6069) -> (-127, 47.6069) projected
  line L32 (-127, 47.6069) -> (-127, 23.8034) projected
  line L33 (-127, 23.8034) -> (-135.89, 23.8034) projected
  line L34 (-135.89, 23.8034) -> (-135.89, -8.89) projected
  line L35 (-135.89, -8.89) -> (-112.8889, -8.89) projected
  line L36 (-112.8889, -8.89) -> (-112.8889, 0) projected
  line L37 (-112.8889, 0) -> (-98.7778, 0) projected
  line L38 (-98.7778, 0) -> (-98.7778, -8.89) projected
  line L39 (-98.7778, -8.89) -> (-84.6667, -8.89) projected
  line L40 (-84.6667, -8.89) -> (-84.6667, 0) projected
  line L41 (-84.6667, 0) -> (-70.5556, 0) projected
  line L42 (-70.5556, 0) -> (-70.5556, -8.89) projected
  line L43 (-70.5556, -8.89) -> (-56.4444, -8.89) projected
  line L44 (-56.4444, -8.89) -> (-56.4444, 0) projected
  line L45 (-56.4444, 0) -> (-42.3333, 0) projected
  line L46 (-42.3333, 0) -> (-42.3333, -8.89) projected
  line L47 (-42.3333, -8.89) -> (-28.2222, -8.89) projected
  line L48 (-28.2222, -8.89) -> (-28.2222, 0) projected
  line L49 (-28.2222, 0) -> (-14.1111, 0) projected
  line L50 (-14.1111, 0) -> (-14.1111, -8.89) projected
  line L51 (-14.1111, -8.89) -> (8.89, -8.89) projected
  line L52 (8.89, -8.89) -> (8.89, 23.8034) projected
  line L53 (8.89, 23.8034) -> (0, 23.8034) projected
  line L54 (0, 23.8034) -> (0, 47.6069) projected
  line L55 (0, 47.6069) -> (8.89, 47.6069) projected
  line L56 (8.89, 47.6069) -> (8.89, 71.4103) projected
  line L57 (8.89, 71.4103) -> (0, 71.4103) projected
  line L58 (0, 71.4103) -> (0, 95.2137) projected
  line L59 (0, 95.2137) -> (8.89, 95.2137) projected
  line L60 (8.89, 95.2137) -> (8.89, 119.0171) projected
  line L61 (8.89, 119.0171) -> (0, 119.0171) projected
  line L62 (0, 119.0171) -> (0, 142.8206) projected
  line L63 (0, 142.8206) -> (8.89, 142.8206) projected
  line L64 (8.89, 142.8206) -> (8.89, 175.514) projected
  line L65 (8.89, 175.514) -> (-14.1111, 175.514) projected
  line L66 (-14.1111, 175.514) -> (-14.1111, 166.624) projected
  line L67 (-14.1111, 166.624) -> (-28.2222, 166.624) projected
  line L68 (-28.2222, 166.624) -> (-28.2222, 175.514) projected
  line L69 (-28.2222, 175.514) -> (-42.3333, 175.514) projected
  line L70 (-42.3333, 175.514) -> (-42.3333, 166.624) projected
  line L71 (-42.3333, 166.624) -> (-56.4444, 166.624) projected
  line L72 (-56.4444, 166.624) -> (-56.4444, 175.514) projected
  line L73 (-56.4444, 175.514) -> (-70.5556, 175.514) projected
  line L74 (-70.5556, 175.514) -> (-70.5556, 166.624) projected
  line L75 (-70.5556, 166.624) -> (-84.6667, 166.624) projected
  line L76 (-84.6667, 166.624) -> (-84.6667, 175.514) projected
  line L77 (-84.6667, 175.514) -> (-98.7778, 175.514) projected
  line L78 (-98.7778, 175.514) -> (-98.7778, 166.624) projected
  line L79 (-98.7778, 166.624) -> (-112.8889, 166.624) projected
  line L80 (-112.8889, 166.624) -> (-112.8889, 175.514) projected
  line L81 (-112.8889, 175.514) -> (-135.89, 175.514) projected
  line L82 (-135.89, 175.514) -> (-135.89, 142.8206) projected
  line L83 (-135.89, 142.8206) -> (-127, 142.8206) projected
  line L84 (-127, 142.8206) -> (-127, 119.0171) projected
  circle A15 centre (-107.555, 112.3994) radius 3.75 projected
  point P0 (0, 0)
sketch "Sketch9" plane through (0, 6.35, 0) normal (0, 1, 0) x (1, 0, 0)
  point P0 (0, 0)
extrude "Extrusion5" cut sketch "Sketch8" against normal blind 25.4 contours L6 L8 L7 L5 L3 L4 L2 L1 L0 | A0 | A1 | A15